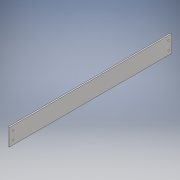
# Autodesk Inventor part: Platte_Kettenglied_unten
Saved by Autodesk Inventor 2018 (Build 220112000, 112)
## iProperties
Created: 2018-01-12
Part Number: Platte_Kettenglied_unten
Material: Generisch
Document SubType Name: Modeling
Designer: Julian
Density: 1 g/cm^3
Appearance: Vorgabe
Author: Julian
Autodesk Inventor part; units mm, degrees
ref_plane "YZ Plane" through (0, 0, 0) normal (1, 0, 0) x (0, 1, 0)
ref_plane "XZ Plane" through (0, 0, 0) normal (0, 1, 0) x (-1, 0, 0)
ref_plane "XY Plane" through (0, 0, 0) normal (0, 0, 1) x (1, 0, 0)
sketch "Skizze1" plane through (0, 0, 0) normal (1, 0, 0) x (0, 1, 0)
  line L0 (0, 0) -> (121.813, 0)
  line L1 (121.813, 0) -> (121.813, 12.7)
  line L2 (121.813, 12.7) -> (0, 12.7)
  line L3 (0, 12.7) -> (0, 0)
  dimension "d0" = 121.813
  dimension "d1" = 12.7
  constraints: 8 end point, 2 parallel, 1 horizontal, 1 perpendicular
  measures "d0" distance of L1.end L2.end
  measures "d1" distance of L0.end L1.end
extrude "Extrusion1" add sketch "Skizze1" along normal blind 1
sketch "Skizze2" plane through (1, 0, 0) normal (1, 0, 0) x (0, 0, -1)
  line L0 (-12.7, 0) -> (0, 0) projected
  line L1 (-6.35, 0) -> (-6.35, 2.5)
  line L2 (-6.35, 2.5) -> (-9.525, 2.5)
  line L3 (-6.35, 2.5) -> (-3.175, 2.5)
  line L4 (0, 121.813) -> (-12.7, 121.813) projected
  line L5 (-6.35, 121.813) -> (-6.35, 119.313)
  line L6 (-6.35, 119.313) -> (-9.525, 119.313)
  line L7 (-6.35, 119.313) -> (-3.175, 119.313)
  dimension "d4" = 2.5
  dimension "d5" = 3.175
  dimension "d6" = 3.175
  dimension "d7" = 2.5
  dimension "d8" = 3.175
  constraints: 12 end point, 2 horizontal, 2 midpoint, 2 perpendicular, 2 vertical
  measures "d4" distance of L1.start L1.end
  measures "d5" distance of L1.end L2.end
  measures "d6" distance of L1.end L3.end
  measures "d7" distance of L5.start L5.end
  measures "d8" distance of L5.end L6.end
hole "Bohrung1" at (1, 2.5, 9.525) at (1, 2.5, 3.175) at (1, 119.313, 9.525) at (1, 119.313, 3.175) direction (-1, 0, 0) diameter 1 end through all
